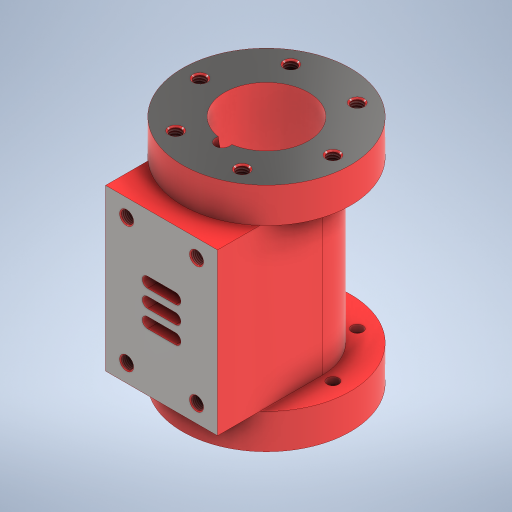
# Autodesk Inventor part: cylinder
Saved by Autodesk Inventor 2023 (Build 270158000, 158)
## iProperties
Created: 2023-10-12
Part Number: cylinder
Material: Ocel, kovaná
Document SubType Name: Modeling
Designer: zak
Density: 7.85 g/cm^3
Appearance: Světle červená
Author: zak
Autodesk Inventor part; units mm, degrees
ref_plane "YZ Plane" through (0, 0, 0) normal (1, 0, 0) x (0, 1, 0)
ref_plane "XY Plane" through (0, 0, 0) normal (0, 0, 1) x (1, 0, 0)
sketch "Náčrt1" plane through (0, 0, 0) normal (1, 0, 0) x (0, 1, 0)
  line L0 (0, -28.8) -> (0, 4.8) projected
  line L1 (-13.2, 0) -> (79.2, 0) projected
  line L2 (0, 0) -> (66, 0)
  line L3 (66, 0) -> (66, -24)
  line L4 (66, -24) -> (56, -24)
  line L5 (56, -24) -> (56, -16)
  line L6 (56, -16) -> (10, -16)
  line L7 (10, -16) -> (10, -24)
  line L8 (10, -24) -> (0, -24)
  line L9 (0, -24) -> (0, 0)
  dimension "d1" = 66
  dimension "d2" = 24
  dimension "d3" = 10
  dimension "d4" = 10
  dimension "d5" = 16
  dimension "d6" = 24
  constraints: 16 end point, 6 perpendicular, 2 point on line, 1 collinear
  measures "d1" distance of L2.start L2.end
  measures "d2" distance of L2.end L3.end
  measures "d3" distance of L3.end L4.end
  measures "d4" distance of L7.end L8.end
  measures "d5" distance between parallel lines of L1 L6
  measures "d6" distance between parallel lines of L1 L8
revolve "Rotace1" add sketch "Náčrt1" angle 360 about axis through (0, -10, 0) along (0, 1, 0)
sketch "Náčrt3" plane through (0, 66, 0) normal (0, 1, 0) x (1, 0, 0)
  circle A0 centre (0, 0) radius 24 construction
  circle A1 centre (0, 0) radius 19 construction
  line L0 (-33.6, 0) -> (33.6, 0) projected
  line L1 (0, 0) -> (-10.3278, 17.8883) construction
  circle A2 centre (0, 0) radius 19 construction
  circle A3 centre (0, 0) radius 19 construction
  circle A4 centre (0, 0) radius 19 construction
  circle A5 centre (0, 0) radius 19 construction
  circle A6 centre (0, 0) radius 19 construction
  point P0 (-9.5, 16.4545)
  point P1 (-19, 0)
  point P2 (-9.5, -16.4545)
  point P3 (9.5, -16.4545)
  point P4 (19, 0)
  point P5 (9.5, 16.4545)
  dimension "d15" = 38
  dimension "d16" = 60
  dimension "d19" = 360
  constraints: 3 coincident, 2 end point, 2 horizontal alignment, 1 point on line, 33 other
  measures "d16" angle of L0 L1
hole "Díra2" at (-9.5, 66, -16.4545) at (-19, 66, 0) at (-9.5, 66, 16.4545) at (9.5, 66, 16.4545) at (19, 66, 0) at (9.5, 66, -16.4545) direction (0, -1, 0) diameter 3.242 depth 10 tip angle 118 countersink diameter 4 countersink angle 90 thread size "M4x0.7" class "6H" standard "ISO Metric profile"
sketch "Náčrt4" plane through (0, 0, 0) normal (0, 0, 1) x (1, 0, 0)
  line L0 (-16, 10) -> (-16, 56) projected
  line L1 (24, 10) -> (-24, 10) projected
  line L2 (-16, 56) -> (16, 56)
  line L3 (16, 56) -> (16, 10)
  line L4 (16, 10) -> (-16, 10)
  line L5 (-16, 10) -> (-16, 56)
  point P0 (0, 0)
  dimension "d28" = 32
  constraints: 8 end point, 2 parallel, 2 point on line, 1 horizontal, 1 perpendicular
  measures "d28" distance of L3.end L4.end
extrude "Vysunutí1" add sketch "Náčrt4" along normal blind 30
sketch "Náčrt2" plane through (0, 66, 0) normal (0, 1, 0) x (1, 0, 0)
  point P0 (0, 0)
  point P1 (0, 0)
  constraints: 1 coincident
hole "Díra1" at (0, 66, 0) direction (0, -1, 0) diameter 24 end through all
sketch "Náčrt5" plane through (0, 0, 30) normal (0, 0, 1) x (1, 0, 0)
  line L0 (0, -13.2) -> (0, 79.2) projected
  line L1 (-16, 10) -> (-16, 56) construction
  line L2 (-16, 33) -> (16.2437, 33) construction
  point P0 (0, 0)
  point P1 (-10, 51)
  point P2 (10, 51)
  dimension "d31" = 10
  constraints: 2 end point, 1 horizontal, 1 midpoint, 1 symmetric about line
  measures "d31" distance from line of L0 point (-10, 51)
hole "Díra3" at (10, 51, 30) at (-10, 51, 30) direction (0, 0, -1) diameter 3.4587 depth 10 tip angle 118 countersink diameter 4 countersink angle 90 thread size "M4x0.5" class "6H" standard "ISO Metric profile"
ref_plane "Pracovní rovina1" through (0, 33, 0) normal (0, 1, 0) x (-1, 0, 0)
sketch "Náčrt7" plane through (0, 0, 30) normal (0, 0, 1) x (1, 0, 0)
  line L0 (-4, 33) -> (4, 33) construction
  line L1 (-4, 31.5) -> (4, 31.5)
  line L2 (4, 34.5) -> (-4, 34.5)
  arc A0 (-4, 34.5) -> (-4, 31.5) centre (-4, 33) ccw
  arc A1 (4, 31.5) -> (4, 34.5) centre (4, 33) ccw
  line L3 (-33.6, 33) -> (33.6, 33) projected
  line L4 (-4, 38) -> (4, 38) construction
  line L5 (-4, 36.5) -> (4, 36.5)
  line L6 (4, 39.5) -> (-4, 39.5)
  arc A2 (-4, 39.5) -> (-4, 36.5) centre (-4, 38) ccw
  arc A3 (4, 36.5) -> (4, 39.5) centre (4, 38) ccw
  line L7 (0, -13.2) -> (0, 79.2) projected
  point P0 (0, 0)
  point P1 (0, 33)
  point P2 (0, 38)
  point P3 (5.5, 33)
  point P4 (-5.5, 33)
  point P5 (0, 39.5)
  point P6 (0, 36.5)
  point P7 (0, 31.5)
  point P8 (0, 34.5)
  dimension "d41" = 4
  dimension "d42" = 3
  dimension "d43" = 4
  dimension "d44" = 3
  dimension "d45" = 2
  constraints: 16 end point, 8 point on circle, 8 tangent, 4 centre point, 3 midpoint, 2 horizontal, 2 parallel, 1 point on line
  measures "d41" distance of point (0, 33) L0.end
  measures "d42" diameter of A1
  measures "d43" distance of point (0, 38) L4.end
  measures "d44" diameter of A3
  measures "d45" distance between parallel lines of L2 L5
extrude "Vysunutí2" cut sketch "Náčrt7" against normal blind 6
sketch "Náčrt6" plane through (0, 0, 0) normal (1, 0, 0) x (0, 1, 0)
  line L0 (33, 40.8) -> (33, -34.8) projected
  line L1 (-13.2, 0) -> (79.2, 0) projected
  line L2 (36.5, 24) -> (39.5, 24) projected
  line L3 (36.5, 30) -> (36.5, 24) projected
  line L4 (39.5, 30) -> (39.5, 24) projected
  line L5 (39.5, 30) -> (36.5, 30) projected
  line L6 (39.5, 30) -> (39.5, 24) projected
  line L7 (39.5, 24) -> (36.5, 24) projected
  line L8 (36.5, 30) -> (36.5, 24) projected
  line L9 (10, 0) -> (56, 0) projected
  line L10 (56, 17.8885) -> (56, 0) projected
  line L11 (56, 17.8885) -> (56, 30) projected
  line L12 (10, 30) -> (56, 30) projected
  line L13 (10, 17.8885) -> (10, 30) projected
  line L14 (10, 0) -> (10, 17.8885) projected
  line L15 (66, -24) -> (66, 24) projected
  line L16 (56, 17.8885) -> (56, 17.8885) projected
  line L17 (56, 17.8885) -> (56, 17.8885) projected
  line L18 (36.5, 24) -> (66, 10.2439)
  line L19 (0, 12) -> (66, 12) projected
  line L20 (36.5, 26.2068) -> (66, 12.4507)
  line L21 (36.5, 30) -> (36.5, 24) projected
  line L22 (36.5, 26.2068) -> (36.5, 24)
  line L23 (66, 12.4507) -> (66, 10.2439)
  point P0 (0, 0)
  point P1 (36.5, 24)
  dimension "d48" = 25
  dimension "d49" = 2
  constraints: 8 end point, 3 point on line, 2 collinear, 1 parallel
  measures "d48" angle of L12 L18
  measures "d49" distance between parallel lines of L18 L20
revolve "Rotace2" cut sketch "Náčrt6" angle 360 about axis through (0, 36.5, 26.2068) along (0, 0.9063078, -0.4226183) contours L20 L4 L2 L3 | L18 L2 L4 L20 L10 | L10 L20 L15 L19 L18 | L19 L15 L18
mirror "Zrcadlit1" about plane through (0, 33, 0) normal (0, 1, 0) of "Rotace2", "Vysunutí2", "Díra3", "Díra1", "Díra2"
sketch "Náčrt8" plane through (-16, 10, 0) normal (-1, 0, 0) x (0, 0, 1)
  line L0 (24, 21.5) -> (24, 24.5) projected
  line L1 (30, 24.5) -> (30, 21.5) projected
  line L2 (30, 24.5) -> (30, 21.5) projected
  line L3 (30, 24.5) -> (24, 24.5) projected
  line L4 (30, 21.5) -> (24, 21.5) projected
  line L5 (24, 24.5) -> (24, 21.5) projected
  line L6 (24, 24.5) -> (24, 21.5) projected
  point P0 (0, -10)
  point P1 (24, 23)
hole "Díra4" at (-16, 33, 24) direction (1, 0, 0) diameter 5.4587 depth 8 countersink diameter 6 countersink angle 90 thread size "M6x0.5" class "6H" standard "ISO Metric profile"
